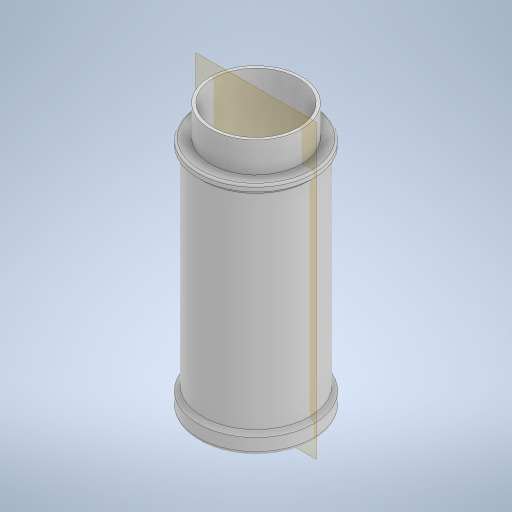
# Autodesk Inventor part: FiestaSpiceContainer
Saved by Autodesk Inventor 2023 (Build 270158000, 158)
## iProperties
Created: 2023-03-20
Part Number: FiestaSpiceContainer
Material: Generic
Document SubType Name: Modeling
Designer: czapa
Density: 1 g/cm^3
Appearance: Default
Author: czapa
Autodesk Inventor part; units mm, degrees
ref_plane "YZ Plane" through (0, 0, 0) normal (1, 0, 0) x (0, 1, 0)
ref_plane "XZ Plane" through (0, 0, 0) normal (0, 1, 0) x (-1, 0, 0)
sketch "Sketch1" plane through (0, 0, 0) normal (0, 1, 0) x (-1, 0, 0)
  circle A0 centre (0, 0) radius 28.5
  dimension "d0" = 57
  constraints: 1 centre point, 1 coincident
  measures "d0" diameter of A0
extrude "Extrusion1" add sketch "Sketch1" along normal blind 131
sketch "Sketch2" plane through (0, 131, 0) normal (0, 1, 0) x (1, 0, 0)
  circle A0 centre (0, 0) radius 25
  circle A1 centre (0, 0) radius 22.5
  circle A2 centre (0, 0) radius 28.5
  dimension "d3" = 50
  dimension "d4" = 45
  dimension "d8" = 57
  constraints: 3 centre point, 3 coincident
  measures "d3" diameter of A0
  measures "d4" diameter of A1
  measures "d8" diameter of A2
extrude "Extrusion2" cut sketch "Sketch2" against normal blind 15 contours A0 | A2
ref_plane "Work Plane2" through (0, 0, 0) normal (0, 0, 1) x (1, 0, 0)
sketch "Sketch4" plane through (0, 0, 0) normal (0, 0, 1) x (1, 0, 0)
  line L0 (28.5, 0) -> (28.5, 116) projected
  line L1 (-28.5, 116) -> (28.5, 116) projected
  line L2 (28.5, 116) -> (28.5, 111)
  line L3 (28.5, 111) -> (26.5, 111)
  line L4 (28.5, 0) -> (-28.5, 0) projected
  line L5 (28.5, 0) -> (28.5, 10)
  line L6 (28.5, 10) -> (26.5, 10)
  line L7 (26.5, 10) -> (26.5, 111)
  line L8 (28.5, 111) -> (28.5, 10)
  line L9 (0, -23.2) -> (0, 139.2) projected
  point P0 (0, 0)
  dimension "d10" = 5
  dimension "d11" = 2
  dimension "d12" = 10
  dimension "d13" = 2
  constraints: 12 end point, 3 point on line, 2 perpendicular, 1 collinear
  measures "d10" distance of L0.end L2.end
  measures "d11" distance of L2.end L3.end
  measures "d12" distance of L0.start L5.end
  measures "d13" distance of L5.end L6.end
revolve "Revolution1" cut sketch "Sketch4" angle 360 about axis through (0, -10, 0) along (0, 1, 0) contours L6 L7 L3 L0
chamfer "Chamfer1" distance 2 angle 45 1 edges at (28.5, 10, 0)
chamfer "Chamfer2" distance 2 angle 45 1 edges at (28.5, 111, 0)
fillet "Fillet1" radius 2 1 edges at (28.5, 0, 0)
fillet "Fillet2" radius 1 1 edges at (28.5, 116, 0)
sketch "Sketch5" plane through (0, 0, 0) normal (0, 0, 1) x (1, 0, 0)
  point P0 (0, 0)
sketch "Sketch6" plane through (0, 131, 0) normal (0, 1, 0) x (1, 0, 0)
  circle A0 centre (0, 0) radius 21
  dimension "d27" = 42
  constraints: 1 centre point, 1 coincident
  measures "d27" diameter of A0
extrude "Extrusion3" cut sketch "Sketch6" against normal blind 125
body "Solid1"
